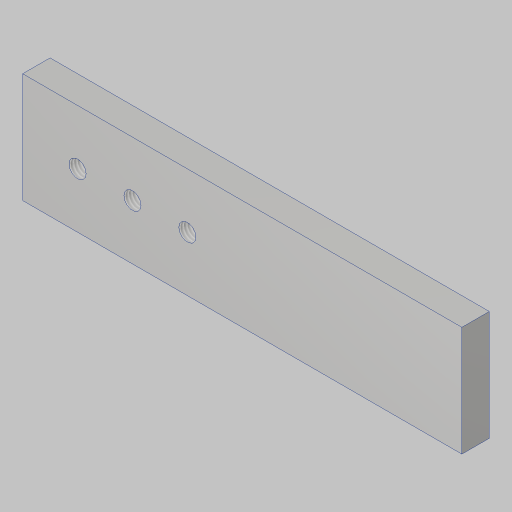
# Autodesk Inventor part: EL2-014
Saved by Autodesk Inventor 2023.5 (Build 275446000, 446)
## iProperties
Created: 2025-01-21
Part Number: EL2-014
Material: Aluminum 6061
Document SubType Name: Modeling
Designer: slick
Density: 2.7 g/cm^3
Appearance: Aluminum - Flat
Author: slick
Autodesk Inventor part; units mm, degrees
ref_plane "YZ Plane" through (0, 0, 0) normal (1, 0, 0) x (0, 1, 0)
ref_plane "XZ Plane" through (0, 0, 0) normal (0, 1, 0) x (-1, 0, 0)
ref_plane "XY Plane" through (0, 0, 0) normal (0, 0, 1) x (1, 0, 0)
sketch "Sketch1" plane through (0, 0, 0) normal (0, 0, 1) x (1, 0, 0)
  line L0 (50.8, -12.7) -> (-50.8, -12.7)
  line L1 (-50.8, -12.7) -> (-50.8, 12.7)
  line L2 (-50.8, 12.7) -> (50.8, 12.7)
  line L3 (50.8, 12.7) -> (50.8, -12.7)
  line L4 (50.8, -12.7) -> (-50.8, 12.7) construction
  line L5 (-50.8, -12.7) -> (50.8, 12.7) construction
  point P0 (0, 0)
  dimension "d0" = 101.6
  dimension "d1" = 25.4
  constraints: 12 end point, 2 midpoint, 2 parallel, 1 horizontal, 1 perpendicular
  measures "d0" distance of L1.end L2.end
  measures "d1" distance of L0.end L1.end
extrude "Extrusion1" add sketch "Sketch1" along normal blind 6.35
sketch "Sketch2" plane through (0, 0, 6.35) normal (0, 0, 1) x (1, 0, 0)
  line L0 (-50.8, 12.7) -> (-50.8, -12.7) projected
  point P0 (0, 0)
  point P1 (-38.1, 0)
  point P2 (-25.4, 0)
  point P3 (-12.7, 0)
  point P4 (-50.8, 0)
  dimension "d4" = 12.7
  dimension "d5" = 12.7
  dimension "d6" = 12.7
  constraints: 1 midpoint
  measures "d4" distance of point (-50.8, 0) point (-38.1, 0)
  measures "d5" distance of point (-25.4, 0) point (-38.1, 0)
  measures "d6" distance of point (-25.4, 0) point (-12.7, 0)
hole "Hole1" at (-38.1, 0, 6.35) at (-25.4, 0, 6.35) at (-12.7, 0, 6.35) direction (0, 0, -1) diameter 3.9624 end through all thread size "10-32 UNF" class "2B" standard "ANSI Unified Screw Threads"
equation "\"d5\" = d4"
equation "\"d6\" = d4"
body "Solid1"
